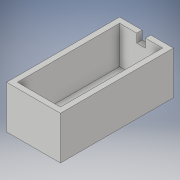
# Autodesk Inventor part: BatteryHolder
Saved by Autodesk Inventor 2017 (Build 210142000, 142)
## iProperties
Created: 2017-03-28
Part Number: BatteryHolder
Material: Generic
Document SubType Name: Modeling
Designer: User
Density: 1 g/cm^3
Appearance: Default
Author: User
Autodesk Inventor part; units mm, degrees
ref_plane "YZ Plane" through (0, 0, 0) normal (1, 0, 0) x (0, 1, 0)
ref_plane "XZ Plane" through (0, 0, 0) normal (0, 1, 0) x (-1, 0, 0)
ref_plane "XY Plane" through (0, 0, 0) normal (0, 0, 1) x (1, 0, 0)
sketch "Sketch1" plane through (0, 0, 0) normal (0, 0, 1) x (1, 0, 0)
  line L0 (0, 0) -> (50.8, 0)
  line L1 (50.8, 0) -> (50.8, 50.8)
  line L2 (50.8, 50.8) -> (0, 50.8)
  line L3 (0, 50.8) -> (0, 0)
  dimension "d0" = 50.8
  dimension "d1" = 50.8
  constraints: 8 end point, 2 parallel, 1 horizontal, 1 perpendicular
  measures "d0" distance of L2.end L1.end
  measures "d1" distance of L1.end L0.end
extrude "Extrusion1" add sketch "Sketch1" along normal blind 6.35
sketch "Sketch2" plane through (0, 50.8, 0) normal (0, 1, 0) x (1, 0, 0)
  line L0 (0, 0) -> (50.8, 0) projected
  line L1 (0, -6.35) -> (50.8, -6.35) projected
  line L2 (20.3299, 0) -> (30.4899, 0)
  line L3 (30.4899, 0) -> (30.4899, -6.35)
  line L4 (30.4899, -6.35) -> (20.3299, -6.35)
  line L5 (20.3299, -6.35) -> (20.3299, 0)
  dimension "d4" = 10.16
  constraints: 8 end point, 2 parallel, 2 point on line, 1 horizontal, 1 perpendicular
  measures "d4" distance of L3.end L4.end
extrude "Extrusion2" cut sketch "Sketch2" against normal blind 10.16
sketch "Sketch3" plane through (50.8, 0, 0) normal (1, 0, 0) x (0, 0, -1)
  line L0 (0, 0) -> (-6.35, 0) projected
  line L1 (0, 0) -> (-133.35, 0)
  line L2 (-133.35, 0) -> (-133.35, 50.8)
  line L3 (-133.35, 50.8) -> (0, 50.8)
  line L4 (0, 50.8) -> (0, 0)
  dimension "d7" = 133.35
  constraints: 8 end point, 2 parallel, 1 horizontal, 1 perpendicular
  measures "d7" distance of L2.end L3.end
extrude "Extrusion3" add sketch "Sketch3" along normal blind 6.35
sketch "Sketch4" plane through (0, 0, 0) normal (-1, 0, 0) x (0, 0, 1)
  line L0 (133.35, 0) -> (133.35, 50.8) projected
  line L1 (0, 0) -> (133.35, 0)
  line L2 (133.35, 0) -> (133.35, 50.8)
  line L3 (133.35, 50.8) -> (0, 50.8)
  line L4 (0, 50.8) -> (0, 0)
  constraints: 8 end point, 2 parallel, 1 horizontal, 1 perpendicular
extrude "Extrusion4" add sketch "Sketch4" along normal blind 6.35
sketch "Sketch5" plane through (0, 0, 0) normal (1, 0, 0) x (0, 0, -1)
  line L0 (-6.35, 0) -> (-133.35, 0) projected
  line L1 (-133.35, 50.8) -> (-6.35, 50.8) projected
  line L2 (-133.35, 0) -> (-127, 0)
  line L3 (-127, 0) -> (-127, 50.8)
  line L4 (-127, 50.8) -> (-133.35, 50.8)
  line L5 (-133.35, 50.8) -> (-133.35, 0)
  point P0 (0, 0)
  dimension "d12" = 6.35
  constraints: 8 end point, 2 parallel, 1 horizontal, 1 perpendicular, 1 point on line
  measures "d12" distance of L4.end L3.end
extrude "Extrusion5" add sketch "Sketch5" along normal blind 50.8
sketch "Sketch6" plane through (57.15, 0, 0) normal (0, -1, 0) x (1, 0, 0)
  line L0 (-57.15, 6.35) -> (-6.35, 6.35) projected
  line L1 (-57.15, 127) -> (-57.15, 6.35) projected
  line L2 (-6.35, 6.35) -> (-57.15, 6.35)
  line L3 (-57.15, 6.35) -> (-57.15, 127)
  line L4 (-57.15, 127) -> (-6.35, 127)
  line L5 (-6.35, 127) -> (-6.35, 6.35)
  point P0 (-57.15, 0)
  constraints: 8 end point, 2 parallel, 1 horizontal, 1 perpendicular
extrude "Extrusion6" add sketch "Sketch6" against normal blind 6.35
equation "\"d5\" = d4"
body "Solid1"
